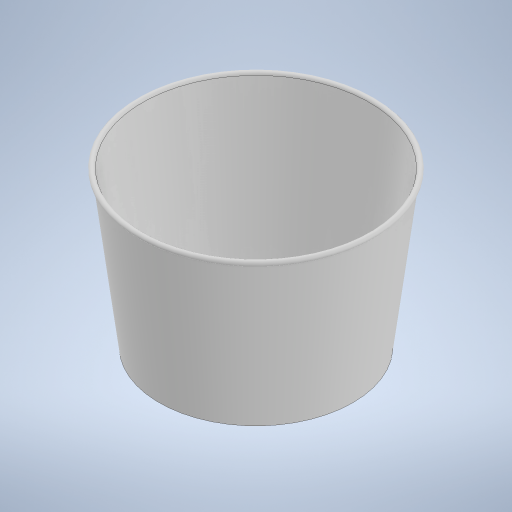
# Autodesk Inventor part: test_2
Saved by Autodesk Inventor 2024.2 (Build 282272000, 272)
## iProperties
Created: 2024-02-28
Part Number: test_2
Material: Genérico
Document SubType Name: Modeling
Designer: riera
Density: 1 g/cm^3
Appearance: Valor por defecto
Author: riera
Autodesk Inventor part; units mm, degrees
ref_plane "YZ Plane" through (0, 0, 0) normal (1, 0, 0) x (0, 1, 0)
ref_plane "XZ Plane" through (0, 0, 0) normal (0, 1, 0) x (-1, 0, 0)
ref_plane "XY Plane" through (0, 0, 0) normal (0, 0, 1) x (1, 0, 0)
sketch "Boceto1" plane through (0, 0, 0) normal (0, 0, 1) x (1, 0, 0)
  line L0 (0, 0) -> (75, 0)
  line L1 (75, 0) -> (89.7517, 118.0136)
  line L2 (87.9844, 120) -> (73.2344, 2)
  line L3 (73.2344, 2) -> (0, 2)
  arc A0 (89.7517, 118.0136) -> (87.9844, 120) centre (89.9844, 120) ccw
  line L4 (0, 2) -> (0, 0)
  line L5 (0, -24.5647) -> (0, 147.3883) projected
  dimension "d0" = 75
  dimension "d3" = 2
  dimension "d4" = 82.875
  dimension "d5" = 4
  constraints: 10 end point, 2 point on circle, 1 centre point, 1 horizontal, 1 vertical
  measures "d0" distance of L0.start L0.end
  measures "d3" distance between parallel lines of L1 L2
  measures "d4" angle of L1 L0
  measures "d5" diameter of A0
revolve "Revolución1" add sketch "Boceto1" angle 360 about axis through (0, -10, 0) along (0, 1, 0)
